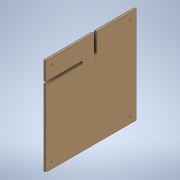
# Autodesk Inventor part: wallL1
Saved by Autodesk Inventor 2022 (Build 260153000, 153)
## iProperties
Created: 2022-02-21
Part Number: wallL1
Material: MDF Medium Density Fiberboard
Document SubType Name: Modeling
Designer: MarkP
Density: 0.8 g/cm^3
Appearance: Cardboard - Corrugated
Author: MarkP
Autodesk Inventor part; units mm, degrees
ref_plane "YZ Plane" through (0, 0, 0) normal (1, 0, 0) x (0, 1, 0)
ref_plane "XZ Plane" through (0, 0, 0) normal (0, 1, 0) x (-1, 0, 0)
ref_plane "XY Plane" through (0, 0, 0) normal (0, 0, 1) x (1, 0, 0)
sketch "Sketch1" plane through (0, 0, 0) normal (1, 0, 0) x (0, 1, 0)
  line L0 (0, 0) -> (800, 0)
  line L1 (800, 0) -> (800, -750)
  line L2 (800, -750) -> (0, -750)
  line L3 (0, -750) -> (0, 0)
  dimension "d0" = 800
  dimension "d1" = 750
  constraints: 8 end point, 2 parallel, 1 horizontal, 1 perpendicular
  measures "d0" distance of L1.end L2.end
  measures "d1" distance of L0.end L1.end
extrude "Extrusion1" add sketch "Sketch1" along normal blind 18
sketch "Sketch2" plane through (18, 0, 0) normal (1, 0, 0) x (0, 0, -1)
  line L0 (0, 800) -> (0, 0) projected
  line L1 (750, 800) -> (0, 800) projected
  line L2 (400, 800) -> (418.5, 800)
  line L3 (418.5, 800) -> (418.5, 650)
  line L4 (418.5, 650) -> (400, 650)
  line L5 (400, 650) -> (400, 800)
  line L6 (0, 650) -> (300, 650)
  line L7 (300, 650) -> (300, 631.5)
  line L8 (300, 631.5) -> (0, 631.5)
  line L9 (0, 631.5) -> (0, 650)
  dimension "d4" = 400
  dimension "d5" = 18.5
  dimension "d6" = 150
  dimension "d7" = 300
  dimension "d8" = 18.5
  constraints: 16 end point, 4 parallel, 2 horizontal, 2 perpendicular, 2 point on line
  measures "d4" distance of L0.start L2.start
  measures "d5" distance of L3.end L4.end
  measures "d6" distance of L2.end L3.end
  measures "d7" distance of L7.end L8.end
  measures "d8" distance of L6.end L7.end
extrude "Extrusion2" cut sketch "Sketch2" against normal blind 18
sketch "Sketch3" plane through (18, 0, 0) normal (1, 0, 0) x (0, 0, -1)
  circle A0 centre (50, 750) radius 5
  circle A1 centre (700, 750) radius 5
  circle A2 centre (700, 50) radius 5
  circle A3 centre (50, 50) radius 5
  point P0 (0, 0)
  point P1 (0, 800)
  constraints: 4 centre point
sketch "Sketch4" plane through (0, 800, -750) normal (0, 1, 0) x (1, 0, 0)
  circle A0 centre (0, -188) radius 5
  circle A1 centre (0, -375) radius 5
  circle A2 centre (0, -562) radius 5
  point P0 (0, -750)
  dimension "d25" = 10
  dimension "d26" = 10
  dimension "d27" = 10
  constraints: 3 centre point
  measures "d25" diameter of A0
  measures "d26" diameter of A1
  measures "d27" diameter of A2
extrude "Extrusion3" cut sketch "Sketch4" against normal blind 32
thread "Thread1" size "M10x1.5" class "6H" standard "ANSI Metric M Profile" full length
thread "Thread2" size "M10x1.5" class "6H" standard "ANSI Metric M Profile" full length
thread "Thread3" size "M10x1.5" class "6H" standard "ANSI Metric M Profile" full length
sketch "Sketch5" plane through (0, 0, -750) normal (0, 0, -1) x (-1, 0, 0)
  line L0 (0, 0) -> (-9, 0)
  line L1 (0, 0) -> (-18, 0) projected
  circle A0 centre (-9, 600) radius 2.5
  circle A1 centre (-9, 200) radius 2.5
  circle A2 centre (-9, 400) radius 2.5
  dimension "d41" = 9
  dimension "d48" = 5
  dimension "d49" = 5
  dimension "d50" = 5
  constraints: 3 centre point, 2 end point, 1 midpoint
  measures "d41" distance of L0.start L0.end
  measures "d48" diameter of A0
  measures "d49" diameter of A1
  measures "d50" diameter of A2
extrude "Extrusion4" cut sketch "Sketch5" against normal blind 18
extrude "Extrusion5" cut sketch "Sketch3" against normal blind 18
sketch "Sketch6" plane through (0, 0, 0) normal (-1, 0, 0) x (0, 0, 1)
  circle A0 centre (-300, 640.75) radius 2.5
  point P0 (0, 0)
  point P1 (-300, 631.5)
  dimension "d56" = 5
  constraints: 1 centre point
  measures "d56" diameter of A0
extrude "Extrusion6" cut sketch "Sketch6" against normal blind 18
sketch "Sketch7" plane through (18, 0, 0) normal (1, 0, 0) x (0, 0, -1)
  point P0 (0, 0)
sketch "Sketch8" plane through (18, 0, 0) normal (1, 0, 0) x (0, 0, -1)
  arc A0 (300, 638.25) -> (300, 643.25) centre (300, 640.75) ccw projected
  line L0 (300, 640.75) -> (409, 640.75) construction
  circle A1 centre (409, 640.75) radius 2.5
  circle A2 centre (409, 590.75) radius 2.5
  point P0 (0, 0)
  dimension "d62" = 5
  dimension "d63" = 5
  constraints: 2 centre point, 2 end point, 1 coincident, 1 horizontal
  measures "d62" diameter of A1
  measures "d63" diameter of A2
extrude "Extrusion7" cut sketch "Sketch8" against normal blind 59.2125
sketch "Sketch9" plane through (18, 0, 0) normal (1, 0, 0) x (0, 0, -1)
  point P0 (0, 0)
body "Solid1"
